Autodesk Fusion 360 part; units mm, degrees
(part 7 of 11)
sketch "Sketch4" plane through (0, 0, 25) normal (0, 0, 1) x (1, 0, 0)
  arc A0 (-57.8411, -108.6864) -> (-56.5947, -103.2256) centre (-92.9957, -97.79) ccw
  arc A1 (-55.7092, -102.5555) -> (-56.5947, -103.2256) centre (-55.8097, -103.3428) ccw
  line L0 (-55.7092, -102.5555) -> (-51.5633, -103.0847)
  spline S0 degree 5 poles (-51.5633, -103.0847) (-51.5364, -103.0882) (-51.4825, -103.0942) (-51.4015, -103.1008) (-51.2932, -103.1049) (-51.1576, -103.1037) (-51.0216, -103.0979) (-50.8855, -103.0894) (-50.7494, -103.0794) (-50.6132, -103.0683) (-50.477, -103.0562) (-50.3407, -103.0425) (-50.2045, -103.0269) (-50.0682, -103.009) (-49.9319, -102.9888) (-49.7956, -102.9666) (-49.6594, -102.9427) (-49.5231, -102.9173) (-49.387, -102.8907) (-49.2509, -102.8628) (-49.1148, -102.8337) (-48.9788, -102.8033) (-48.8429, -102.7715) (-48.7071, -102.7383) (-48.5714, -102.7037) (-48.4357, -102.6678) (-48.3001, -102.6307) (-48.1647, -102.5924) (-48.0293, -102.5529) (-47.8941, -102.5123) (-47.759, -102.4706) (-47.624, -102.4278) (-47.4891, -102.3838) (-47.3544, -102.3388) (-47.2198, -102.2926) (-47.0853, -102.2454) (-46.9509, -102.1971) (-46.8168, -102.1477) (-46.6827, -102.0974) (-46.5488, -102.046) (-46.4151, -101.9936) (-46.2815, -101.9403) (-46.1481, -101.886) (-46.0149, -101.8306) (-45.8818, -101.7744) (-45.7489, -101.7171) (-45.6162, -101.659) (-45.4836, -101.5999) (-45.3513, -101.5398) (-45.2191, -101.4789) (-45.0871, -101.417) (-44.9553, -101.3543) (-44.8237, -101.2906) (-44.6923, -101.2261) (-44.5611, -101.1607) (-44.4302, -101.0944) (-44.2994, -101.0273) (-44.1688, -100.9593) (-44.0384, -100.8904) (-43.9083, -100.8207) (-43.7783, -100.7502) (-43.6486, -100.6788) (-43.5191, -100.6067) (-43.3899, -100.5336) (-43.2608, -100.4598) (-43.132, -100.3852) (-43.0035, -100.3098) (-42.8751, -100.2335) (-42.747, -100.1565) (-42.6192, -100.0787) (-42.4916, -100.0001) (-42.3897, -99.9366) (-42.3133, -99.8886) (-42.2625, -99.8565) (-42.2371, -99.8404) knots 0 0 0 0 0 0 0.01428571 0.02857143 0.04285714 0.05714286 0.07142857 0.08571429 0.1 0.11428571 0.12857143 0.14285714 0.15714286 0.17142857 0.18571429 0.2 0.21428571 0.22857143 0.24285714 0.25714286 0.27142857 0.28571429 0.3 0.31428571 0.32857143 0.34285714 0.35714286 0.37142857 0.38571429 0.4 0.41428571 0.42857143 0.44285714 0.45714286 0.47142857 0.48571429 0.5 0.51428571 0.52857143 0.54285714 0.55714286 0.57142857 0.58571429 0.6 0.61428571 0.62857143 0.64285714 0.65714286 0.67142857 0.68571429 0.7 0.71428571 0.72857143 0.74285714 0.75714286 0.77142857 0.78571429 0.8 0.81428571 0.82857143 0.84285714 0.85714286 0.87142857 0.88571429 0.9 0.91428571 0.92857143 0.94285714 0.95714286 0.97142857 0.98571429 1 1 1 1 1 1
  arc A2 (-42.2371, -99.8404) -> (-42.2371, -95.7395) centre (-92.9957, -97.79) ccw
  spline S1 degree 5 poles (-42.2371, -95.7395) (-42.2625, -95.7234) (-42.3133, -95.6913) (-42.3897, -95.6433) (-42.4916, -95.5798) (-42.6192, -95.5012) (-42.747, -95.4234) (-42.8751, -95.3464) (-43.0035, -95.2702) (-43.132, -95.1947) (-43.2608, -95.1201) (-43.3899, -95.0463) (-43.5191, -94.9733) (-43.6486, -94.9011) (-43.7783, -94.8297) (-43.9083, -94.7592) (-44.0384, -94.6895) (-44.1688, -94.6206) (-44.2994, -94.5526) (-44.4302, -94.4855) (-44.5611, -94.4192) (-44.6923, -94.3538) (-44.8237, -94.2893) (-44.9553, -94.2256) (-45.0871, -94.1629) (-45.2191, -94.101) (-45.3513, -94.0401) (-45.4836, -93.9801) (-45.6162, -93.9209) (-45.7489, -93.8628) (-45.8818, -93.8055) (-46.0149, -93.7493) (-46.1481, -93.694) (-46.2815, -93.6396) (-46.4151, -93.5863) (-46.5488, -93.5339) (-46.6827, -93.4825) (-46.8168, -93.4322) (-46.9509, -93.3829) (-47.0853, -93.3346) (-47.2198, -93.2873) (-47.3544, -93.2411) (-47.4891, -93.1961) (-47.624, -93.1521) (-47.759, -93.1093) (-47.8941, -93.0676) (-48.0293, -93.027) (-48.1647, -92.9875) (-48.3001, -92.9492) (-48.4357, -92.9121) (-48.5714, -92.8762) (-48.7071, -92.8416) (-48.8429, -92.8084) (-48.9788, -92.7766) (-49.1148, -92.7462) (-49.2509, -92.7171) (-49.387, -92.6892) (-49.5231, -92.6626) (-49.6594, -92.6372) (-49.7956, -92.6133) (-49.9319, -92.5911) (-50.0682, -92.5709) (-50.2045, -92.553) (-50.3407, -92.5374) (-50.477, -92.5237) (-50.6132, -92.5116) (-50.7494, -92.5005) (-50.8855, -92.4905) (-51.0216, -92.482) (-51.1576, -92.4762) (-51.2932, -92.475) (-51.4015, -92.4791) (-51.4825, -92.4857) (-51.5364, -92.4917) (-51.5633, -92.4952) knots -1 -1 -1 -1 -1 -1 -0.98571429 -0.97142857 -0.95714286 -0.94285714 -0.92857143 -0.91428571 -0.9 -0.88571429 -0.87142857 -0.85714286 -0.84285714 -0.82857143 -0.81428571 -0.8 -0.78571429 -0.77142857 -0.75714286 -0.74285714 -0.72857143 -0.71428571 -0.7 -0.68571429 -0.67142857 -0.65714286 -0.64285714 -0.62857143 -0.61428571 -0.6 -0.58571429 -0.57142857 -0.55714286 -0.54285714 -0.52857143 -0.51428571 -0.5 -0.48571429 -0.47142857 -0.45714286 -0.44285714 -0.42857143 -0.41428571 -0.4 -0.38571429 -0.37142857 -0.35714286 -0.34285714 -0.32857143 -0.31428571 -0.3 -0.28571429 -0.27142857 -0.25714286 -0.24285714 -0.22857143 -0.21428571 -0.2 -0.18571429 -0.17142857 -0.15714286 -0.14285714 -0.12857143 -0.11428571 -0.1 -0.08571429 -0.07142857 -0.05714286 -0.04285714 -0.02857143 -0.01428571 0 0 0 0 0 0
  line L1 (-51.5633, -92.4952) -> (-55.7092, -93.0245)
  arc A3 (-56.5947, -92.3543) -> (-55.7092, -93.0245) centre (-55.8097, -92.2371) ccw
  arc A4 (-56.5947, -92.3543) -> (-57.8411, -86.8935) centre (-92.9957, -97.79) ccw
  arc A5 (-57.334, -85.9055) -> (-57.8411, -86.8935) centre (-57.083, -86.6585) ccw
  line L2 (-57.334, -85.9055) -> (-53.3691, -84.5835)
  spline S2 degree 5 poles (-53.3691, -84.5835) (-53.3434, -84.575) (-53.2922, -84.557) (-53.2163, -84.5278) (-53.117, -84.4846) (-52.9953, -84.4246) (-52.8753, -84.3604) (-52.7564, -84.2937) (-52.6381, -84.2256) (-52.5202, -84.1565) (-52.4027, -84.0865) (-52.2859, -84.0151) (-52.1699, -83.9418) (-52.0549, -83.8666) (-51.9409, -83.7893) (-51.8277, -83.7102) (-51.7153, -83.6295) (-51.6036, -83.5475) (-51.4925, -83.4644) (-51.3819, -83.3803) (-51.272, -83.295) (-51.1627, -83.2086) (-51.054, -83.121) (-50.9461, -83.0321) (-50.8388, -82.9421) (-50.7321, -82.8509) (-50.6261, -82.7586) (-50.5207, -82.6653) (-50.4158, -82.5711) (-50.3116, -82.4758) (-50.208, -82.3796) (-50.1049, -82.2824) (-50.0025, -82.1843) (-49.9006, -82.0853) (-49.7994, -81.9853) (-49.6987, -81.8843) (-49.5986, -81.7825) (-49.4991, -81.6799) (-49.4002, -81.5763) (-49.3019, -81.472) (-49.2041, -81.3668) (-49.1069, -81.2608) (-49.0103, -81.1539) (-48.9143, -81.0463) (-48.8188, -80.9378) (-48.7239, -80.8286) (-48.6295, -80.7186) (-48.5358, -80.6078) (-48.4426, -80.4963) (-48.3499, -80.3841) (-48.2578, -80.2711) (-48.1663, -80.1574) (-48.0754, -80.0429) (-47.985, -79.9278) (-47.8952, -79.8119) (-47.8059, -79.6954) (-47.7172, -79.5781) (-47.6291, -79.4602) (-47.5415, -79.3416) (-47.4545, -79.2224) (-47.368, -79.1024) (-47.2821, -78.9819) (-47.1967, -78.8606) (-47.112, -78.7388) (-47.0277, -78.6163) (-46.9441, -78.4931) (-46.8609, -78.3694) (-46.7784, -78.245) (-46.6964, -78.1201) (-46.615, -77.9945) (-46.5341, -77.8683) (-46.4698, -77.7669) (-46.4219, -77.6905) (-46.39, -77.6395) (-46.3741, -77.614) knots 0 0 0 0 0 0 0.01428571 0.02857143 0.04285714 0.05714286 0.07142857 0.08571429 0.1 0.11428571 0.12857143 0.14285714 0.15714286 0.17142857 0.18571429 0.2 0.21428571 0.22857143 0.24285714 0.25714286 0.27142857 0.28571429 0.3 0.31428571 0.32857143 0.34285714 0.35714286 0.37142857 0.38571429 0.4 0.41428571 0.42857143 0.44285714 0.45714286 0.47142857 0.48571429 0.5 0.51428571 0.52857143 0.54285714 0.55714286 0.57142857 0.58571429 0.6 0.61428571 0.62857143 0.64285714 0.65714286 0.67142857 0.68571429 0.7 0.71428571 0.72857143 0.74285714 0.75714286 0.77142857 0.78571429 0.8 0.81428571 0.82857143 0.84285714 0.85714286 0.87142857 0.88571429 0.9 0.91428571 0.92857143 0.94285714 0.95714286 0.97142857 0.98571429 1 1 1 1 1 1
  arc A6 (-46.3741, -77.614) -> (-48.1534, -73.9192) centre (-92.9957, -97.79) ccw
  spline S3 degree 5 poles (-48.1534, -73.9192) (-48.1833, -73.9158) (-48.2431, -73.9089) (-48.3326, -73.8987) (-48.452, -73.8857) (-48.6011, -73.8703) (-48.75, -73.8557) (-48.8988, -73.8419) (-49.0475, -73.8289) (-49.1961, -73.8167) (-49.3445, -73.8053) (-49.4928, -73.7948) (-49.641, -73.7851) (-49.789, -73.7763) (-49.9368, -73.7682) (-50.0845, -73.7611) (-50.232, -73.7547) (-50.3793, -73.7493) (-50.5264, -73.7447) (-50.6734, -73.7409) (-50.8202, -73.738) (-50.9668, -73.736) (-51.1132, -73.7349) (-51.2593, -73.7347) (-51.4053, -73.7353) (-51.5511, -73.7369) (-51.6966, -73.7393) (-51.8419, -73.7426) (-51.9869, -73.7469) (-52.1318, -73.7521) (-52.2763, -73.7582) (-52.4206, -73.7652) (-52.5647, -73.7732) (-52.7085, -73.7821) (-52.8519, -73.792) (-52.9951, -73.8028) (-53.1381, -73.8147) (-53.2807, -73.8274) (-53.423, -73.8412) (-53.565, -73.856) (-53.7066, -73.8718) (-53.8479, -73.8886) (-53.9889, -73.9064) (-54.1295, -73.9254) (-54.2697, -73.9453) (-54.4095, -73.9664) (-54.549, -73.9885) (-54.6881, -74.0117) (-54.8267, -74.0359) (-54.965, -74.0613) (-55.1028, -74.0878) (-55.2401, -74.1155) (-55.3768, -74.1446) (-55.5131, -74.1749) (-55.6488, -74.2065) (-55.784, -74.2393) (-55.9187, -74.2732) (-56.053, -74.3083) (-56.1867, -74.3446) (-56.3198, -74.3821) (-56.4523, -74.4213) (-56.5838, -74.4622) (-56.7144, -74.5052) (-56.8439, -74.5502) (-56.9726, -74.597) (-57.1006, -74.6452) (-57.2281, -74.6943) (-57.3551, -74.7444) (-57.4814, -74.7958) (-57.6064, -74.8496) (-57.7292, -74.9073) (-57.8249, -74.958) (-57.895, -74.9991) (-57.941, -75.0279) (-57.9637, -75.0427) knots -1 -1 -1 -1 -1 -1 -0.98571429 -0.97142857 -0.95714286 -0.94285714 -0.92857143 -0.91428571 -0.9 -0.88571429 -0.87142857 -0.85714286 -0.84285714 -0.82857143 -0.81428571 -0.8 -0.78571429 -0.77142857 -0.75714286 -0.74285714 -0.72857143 -0.71428571 -0.7 -0.68571429 -0.67142857 -0.65714286 -0.64285714 -0.62857143 -0.61428571 -0.6 -0.58571429 -0.57142857 -0.55714286 -0.54285714 -0.52857143 -0.51428571 -0.5 -0.48571429 -0.47142857 -0.45714286 -0.44285714 -0.42857143 -0.41428571 -0.4 -0.38571429 -0.37142857 -0.35714286 -0.34285714 -0.32857143 -0.31428571 -0.3 -0.28571429 -0.27142857 -0.25714286 -0.24285714 -0.22857143 -0.21428571 -0.2 -0.18571429 -0.17142857 -0.15714286 -0.14285714 -0.12857143 -0.11428571 -0.1 -0.08571429 -0.07142857 -0.05714286 -0.04285714 -0.02857143 -0.01428571 0 0 0 0 0 0
  line L3 (-57.9637, -75.0427) -> (-61.4694, -77.3184)
  arc A7 (-62.558, -77.0988) -> (-61.4694, -77.3184) centre (-61.9015, -76.6526) ccw
  arc A8 (-62.558, -77.0988) -> (-66.0503, -72.7196) centre (-92.9957, -97.79) ccw
  arc A9 (-66.0221, -71.6094) -> (-66.0503, -72.7196) centre (-65.4692, -72.1789) ccw
  line L4 (-66.0221, -71.6094) -> (-63.0234, -68.698)
  spline S4 degree 5 poles (-63.0234, -68.698) (-63.0039, -68.6791) (-62.9656, -68.6408) (-62.9099, -68.5816) (-62.8392, -68.4995) (-62.7556, -68.3926) (-62.6754, -68.2827) (-62.5972, -68.171) (-62.5201, -68.0583) (-62.4438, -67.945) (-62.3684, -67.8309) (-62.2941, -67.7159) (-62.2214, -67.5996) (-62.1505, -67.4819) (-62.0812, -67.3627) (-62.0136, -67.2424) (-61.9474, -67.1209) (-61.8823, -66.9986) (-61.8182, -66.8755) (-61.7551, -66.7517) (-61.6931, -66.6272) (-61.6321, -66.5019) (-61.5722, -66.3759) (-61.5135, -66.249) (-61.4558, -66.1213) (-61.3993, -65.9928) (-61.3438, -65.8637) (-61.2893, -65.7339) (-61.2358, -65.6035) (-61.1832, -65.4724) (-61.1316, -65.3408) (-61.0809, -65.2085) (-61.0312, -65.0757) (-60.9824, -64.9422) (-60.9346, -64.8082) (-60.8877, -64.6736) (-60.8417, -64.5385) (-60.7966, -64.4028) (-60.7524, -64.2666) (-60.709, -64.1299) (-60.6666, -63.9927) (-60.625, -63.855) (-60.5843, -63.7168) (-60.5445, -63.5782) (-60.5055, -63.4391) (-60.4674, -63.2995) (-60.4302, -63.1594) (-60.3937, -63.019) (-60.3581, -62.878) (-60.3234, -62.7367) (-60.2894, -62.595) (-60.2563, -62.4528) (-60.224, -62.3102) (-60.1926, -62.1673) (-60.1619, -62.0239) (-60.132, -61.8802) (-60.103, -61.7361) (-60.0747, -61.5916) (-60.0473, -61.4467) (-60.0206, -61.3015) (-59.9948, -61.1559) (-59.9697, -61.01) (-59.9454, -60.8638) (-59.9219, -60.7172) (-59.8991, -60.5703) (-59.8772, -60.423) (-59.856, -60.2755) (-59.8356, -60.1276) (-59.8159, -59.9795) (-59.797, -59.831) (-59.7789, -59.6822) (-59.765, -59.563) (-59.755, -59.4734) (-59.7484, -59.4136) (-59.7452, -59.3837) knots 0 0 0 0 0 0 0.01428571 0.02857143 0.04285714 0.05714286 0.07142857 0.08571429 0.1 0.11428571 0.12857143 0.14285714 0.15714286 0.17142857 0.18571429 0.2 0.21428571 0.22857143 0.24285714 0.25714286 0.27142857 0.28571429 0.3 0.31428571 0.32857143 0.34285714 0.35714286 0.37142857 0.38571429 0.4 0.41428571 0.42857143 0.44285714 0.45714286 0.47142857 0.48571429 0.5 0.51428571 0.52857143 0.54285714 0.55714286 0.57142857 0.58571429 0.6 0.61428571 0.62857143 0.64285714 0.65714286 0.67142857 0.68571429 0.7 0.71428571 0.72857143 0.74285714 0.75714286 0.77142857 0.78571429 0.8 0.81428571 0.82857143 0.84285714 0.85714286 0.87142857 0.88571429 0.9 0.91428571 0.92857143 0.94285714 0.95714286 0.97142857 0.98571429 1 1 1 1 1 1
  arc A10 (-59.7452, -59.3837) -> (-62.9513, -56.8269) centre (-92.9957, -97.79) ccw
  spline S5 degree 5 poles (-62.9513, -56.8269) (-62.9798, -56.8367) (-63.0366, -56.8564) (-63.1217, -56.8861) (-63.2349, -56.9262) (-63.3759, -56.977) (-63.5164, -57.0284) (-63.6565, -57.0806) (-63.7961, -57.1334) (-63.9352, -57.1869) (-64.0739, -57.241) (-64.2121, -57.2959) (-64.3498, -57.3514) (-64.4869, -57.4077) (-64.6236, -57.4646) (-64.7598, -57.5222) (-64.8954, -57.5805) (-65.0305, -57.6395) (-65.1651, -57.6992) (-65.2991, -57.7596) (-65.4326, -57.8207) (-65.5656, -57.8824) (-65.6979, -57.9449) (-65.8297, -58.0082) (-65.961, -58.0721) (-66.0916, -58.1367) (-66.2217, -58.202) (-66.3511, -58.2681) (-66.48, -58.3349) (-66.6082, -58.4024) (-66.7358, -58.4706) (-66.8628, -58.5395) (-66.9891, -58.6092) (-67.1148, -58.6796) (-67.2398, -58.7508) (-67.3641, -58.8227) (-67.4877, -58.8954) (-67.6106, -58.9688) (-67.7329, -59.0429) (-67.8544, -59.1178) (-67.9752, -59.1935) (-68.0952, -59.27) (-68.2145, -59.3472) (-68.3329, -59.4253) (-68.4506, -59.5041) (-68.5674, -59.5837) (-68.6835, -59.6642) (-68.7987, -59.7454) (-68.9131, -59.8274) (-69.0267, -59.9102) (-69.1393, -59.9939) (-69.251, -60.0785) (-69.3616, -60.164) (-69.4712, -60.2504) (-69.5798, -60.3378) (-69.6874, -60.426) (-69.794, -60.515) (-69.8997, -60.6049) (-70.0045, -60.6955) (-70.1082, -60.7872) (-70.2105, -60.8799) (-70.3112, -60.9739) (-70.4102, -61.0692) (-70.5074, -61.166) (-70.603, -61.264) (-70.6974, -61.3629) (-70.791, -61.4625) (-70.8837, -61.5628) (-70.9752, -61.6638) (-71.0645, -61.7665) (-71.1501, -61.8718) (-71.2143, -61.959) (-71.2597, -62.0265) (-71.2886, -62.0724) (-71.3027, -62.0956) knots -1 -1 -1 -1 -1 -1 -0.98571429 -0.97142857 -0.95714286 -0.94285714 -0.92857143 -0.91428571 -0.9 -0.88571429 -0.87142857 -0.85714286 -0.84285714 -0.82857143 -0.81428571 -0.8 -0.78571429 -0.77142857 -0.75714286 -0.74285714 -0.72857143 -0.71428571 -0.7 -0.68571429 -0.67142857 -0.65714286 -0.64285714 -0.62857143 -0.61428571 -0.6 -0.58571429 -0.57142857 -0.55714286 -0.54285714 -0.52857143 -0.51428571 -0.5 -0.48571429 -0.47142857 -0.45714286 -0.44285714 -0.42857143 -0.41428571 -0.4 -0.38571429 -0.37142857 -0.35714286 -0.34285714 -0.32857143 -0.31428571 -0.3 -0.28571429 -0.27142857 -0.25714286 -0.24285714 -0.22857143 -0.21428571 -0.2 -0.18571429 -0.17142857 -0.15714286 -0.14285714 -0.12857143 -0.11428571 -0.1 -0.08571429 -0.07142857 -0.05714286 -0.04285714 -0.02857143 -0.01428571 0 0 0 0 0 0
  line L5 (-71.3027, -62.0956) -> (-73.4737, -65.6669)
  arc A11 (-74.5498, -65.9415) -> (-73.4737, -65.6669) centre (-74.152, -65.2546) ccw
  arc A12 (-74.5498, -65.9415) -> (-79.5964, -63.5111) centre (-92.9957, -97.79) ccw
  arc A13 (-80.0527, -62.4987) -> (-79.5964, -63.5111) centre (-79.3074, -62.7719) ccw
  line L6 (-80.0527, -62.4987) -> (-78.6141, -58.5746)
  spline S6 degree 5 poles (-78.6141, -58.5746) (-78.6048, -58.5491) (-78.5869, -58.4979) (-78.5624, -58.4204) (-78.5343, -58.3157) (-78.5053, -58.1832) (-78.4807, -58.0494) (-78.4588, -57.9148) (-78.4382, -57.7798) (-78.4187, -57.6446) (-78.4002, -57.5091) (-78.3832, -57.3732) (-78.3681, -57.2369) (-78.3553, -57.1001) (-78.3446, -56.9627) (-78.3359, -56.8249) (-78.3289, -56.6867) (-78.3234, -56.5483) (-78.319, -56.4096) (-78.3159, -56.2707) (-78.314, -56.1316) (-78.3134, -55.9922) (-78.3142, -55.8527) (-78.3163, -55.7129) (-78.3198, -55.5728) (-78.3246, -55.4326) (-78.3306, -55.2922) (-78.3379, -55.1516) (-78.3462, -55.0108) (-78.3557, -54.87) (-78.3663, -54.7289) (-78.378, -54.5878) (-78.3908, -54.4465) (-78.4048, -54.3051) (-78.4199, -54.1636) (-78.436, -54.022) (-78.4532, -53.8803) (-78.4714, -53.7385) (-78.4907, -53.5966) (-78.511, -53.4546) (-78.5323, -53.3126) (-78.5546, -53.1705) (-78.5778, -53.0284) (-78.6021, -52.8862) (-78.6274, -52.7439) (-78.6536, -52.6016) (-78.6808, -52.4593) (-78.7089, -52.3169) (-78.738, -52.1745) (-78.768, -52.0321) (-78.7989, -51.8896) (-78.8308, -51.7472) (-78.8635, -51.6047) (-78.8972, -51.4623) (-78.9318, -51.3198) (-78.9672, -51.1773) (-79.0036, -51.0349) (-79.0408, -50.8925) (-79.079, -50.75) (-79.1179, -50.6076) (-79.1578, -50.4653) (-79.1985, -50.3229) (-79.2401, -50.1806) (-79.2825, -50.0384) (-79.3257, -49.8961) (-79.3698, -49.7539) (-79.4148, -49.6118) (-79.4605, -49.4697) (-79.5071, -49.3277) (-79.5545, -49.1857) (-79.6027, -49.0438) (-79.642, -48.9304) (-79.6718, -48.8453) (-79.6918, -48.7886) (-79.7018, -48.7602) knots 0 0 0 0 0 0 0.01428571 0.02857143 0.04285714 0.05714286 0.07142857 0.08571429 0.1 0.11428571 0.12857143 0.14285714 0.15714286 0.17142857 0.18571429 0.2 0.21428571 0.22857143 0.24285714 0.25714286 0.27142857 0.28571429 0.3 0.31428571 0.32857143 0.34285714 0.35714286 0.37142857 0.38571429 0.4 0.41428571 0.42857143 0.44285714 0.45714286 0.47142857 0.48571429 0.5 0.51428571 0.52857143 0.54285714 0.55714286 0.57142857 0.58571429 0.6 0.61428571 0.62857143 0.64285714 0.65714286 0.67142857 0.68571429 0.7 0.71428571 0.72857143 0.74285714 0.75714286 0.77142857 0.78571429 0.8 0.81428571 0.82857143 0.84285714 0.85714286 0.87142857 0.88571429 0.9 0.91428571 0.92857143 0.94285714 0.95714286 0.97142857 0.98571429 1 1 1 1 1 1
  arc A14 (-79.7018, -48.7602) -> (-83.6999, -47.8477) centre (-92.9957, -97.79) ccw
  spline S7 degree 5 poles (-83.6999, -47.8477) (-83.7212, -47.8689) (-83.7639, -47.9113) (-83.8276, -47.975) (-83.9122, -48.0602) (-84.0172, -48.1672) (-84.1215, -48.2745) (-84.2251, -48.3822) (-84.328, -48.4904) (-84.4302, -48.599) (-84.5316, -48.7079) (-84.6323, -48.8173) (-84.7322, -48.9271) (-84.8314, -49.0373) (-84.9299, -49.1478) (-85.0275, -49.2588) (-85.1244, -49.3702) (-85.2206, -49.482) (-85.3159, -49.5942) (-85.4105, -49.7067) (-85.5042, -49.8197) (-85.5972, -49.933) (-85.6894, -50.0468) (-85.7807, -50.1609) (-85.8712, -50.2754) (-85.9609, -50.3903) (-86.0497, -50.5056) (-86.1377, -50.6213) (-86.2248, -50.7374) (-86.311, -50.8538) (-86.3964, -50.9707) (-86.4809, -51.0879) (-86.5645, -51.2055) (-86.6471, -51.3235) (-86.7288, -51.4418) (-86.8097, -51.5605) (-86.8895, -51.6796) (-86.9684, -51.7991) (-87.0464, -51.9189) (-87.1234, -52.0392) (-87.1994, -52.1598) (-87.2743, -52.2807) (-87.3482, -52.4021) (-87.4211, -52.5238) (-87.4929, -52.6459) (-87.5636, -52.7683) (-87.6333, -52.8911) (-87.7019, -53.0143) (-87.7694, -53.1378) (-87.8358, -53.2617) (-87.9009, -53.386) (-87.9649, -53.5106) (-88.0274, -53.6357) (-88.0887, -53.7611) (-88.1486, -53.8869) (-88.2072, -54.013) (-88.2647, -54.1395) (-88.321, -54.2664) (-88.376, -54.3935) (-88.4297, -54.5211) (-88.4816, -54.649) (-88.5316, -54.7774) (-88.5794, -54.9063) (-88.625, -55.0356) (-88.6686, -55.1654) (-88.7108, -55.2955) (-88.7518, -55.4258) (-88.7919, -55.5563) (-88.8305, -55.6871) (-88.8664, -55.8184) (-88.8978, -55.9504) (-88.9178, -56.0568) (-88.9294, -56.1372) (-88.9355, -56.1911) (-88.9382, -56.2182) knots -1 -1 -1 -1 -1 -1 -0.98571429 -0.97142857 -0.95714286 -0.94285714 -0.92857143 -0.91428571 -0.9 -0.88571429 -0.87142857 -0.85714286 -0.84285714 -0.82857143 -0.81428571 -0.8 -0.78571429 -0.77142857 -0.75714286 -0.74285714 -0.72857143 -0.71428571 -0.7 -0.68571429 -0.67142857 -0.65714286 -0.64285714 -0.62857143 -0.61428571 -0.6 -0.58571429 -0.57142857 -0.55714286 -0.54285714 -0.52857143 -0.51428571 -0.5 -0.48571429 -0.47142857 -0.45714286 -0.44285714 -0.42857143 -0.41428571 -0.4 -0.38571429 -0.37142857 -0.35714286 -0.34285714 -0.32857143 -0.31428571 -0.3 -0.28571429 -0.27142857 -0.25714286 -0.24285714 -0.22857143 -0.21428571 -0.2 -0.18571429 -0.17142857 -0.15714286 -0.14285714 -0.12857143 -0.11428571 -0.1 -0.08571429 -0.07142857 -0.05714286 -0.04285714 -0.02857143 -0.01428571 0 0 0 0 0 0
  line L7 (-88.9382, -56.2182) -> (-89.3447, -60.3778)
  arc A15 (-90.1951, -61.0921) -> (-89.3447, -60.3778) centre (-90.1347, -60.3006) ccw
  arc A16 (-90.1951, -61.0921) -> (-95.7964, -61.0921) centre (-92.9957, -97.79) ccw
  arc A17 (-96.6467, -60.3778) -> (-95.7964, -61.0921) centre (-95.8568, -60.3006) ccw
  line L8 (-96.6467, -60.3778) -> (-97.0533, -56.2182)
  spline S8 degree 5 poles (-97.0533, -56.2182) (-97.0559, -56.1911) (-97.062, -56.1372) (-97.0736, -56.0568) (-97.0937, -55.9504) (-97.1251, -55.8184) (-97.161, -55.6871) (-97.1996, -55.5563) (-97.2396, -55.4258) (-97.2807, -55.2955) (-97.3228, -55.1654) (-97.3665, -55.0356) (-97.412, -54.9063) (-97.4598, -54.7774) (-97.5098, -54.649) (-97.5618, -54.5211) (-97.6154, -54.3935) (-97.6705, -54.2664) (-97.7268, -54.1395) (-97.7842, -54.013) (-97.8428, -53.8869) (-97.9028, -53.7611) (-97.964, -53.6357) (-98.0266, -53.5106) (-98.0905, -53.386) (-98.1557, -53.2617) (-98.222, -53.1378) (-98.2895, -53.0143) (-98.3581, -52.8911) (-98.4278, -52.7683) (-98.4985, -52.6459) (-98.5703, -52.5238) (-98.6432, -52.4021) (-98.7171, -52.2807) (-98.7921, -52.1598) (-98.8681, -52.0392) (-98.945, -51.9189) (-99.023, -51.7991) (-99.1019, -51.6796) (-99.1818, -51.5605) (-99.2626, -51.4418) (-99.3443, -51.3235) (-99.427, -51.2055) (-99.5106, -51.0879) (-99.595, -50.9707) (-99.6804, -50.8538) (-99.7666, -50.7374) (-99.8538, -50.6213) (-99.9417, -50.5056) (-100.0306, -50.3903) (-100.1202, -50.2754) (-100.2107, -50.1609) (-100.3021, -50.0468) (-100.3942, -49.933) (-100.4872, -49.8197) (-100.581, -49.7067) (-100.6755, -49.5942) (-100.7709, -49.482) (-100.867, -49.3702) (-100.9639, -49.2588) (-101.0616, -49.1478) (-101.16, -49.0373) (-101.2592, -48.9271) (-101.3592, -48.8173) (-101.4599, -48.7079) (-101.5613, -48.599) (-101.6634, -48.4904) (-101.7663, -48.3822) (-101.8699, -48.2745) (-101.9742, -48.1672) (-102.0792, -48.0602) (-102.1638, -47.975) (-102.2275, -47.9113) (-102.2702, -47.8689) (-102.2915, -47.8477) knots 0 0 0 0 0 0 0.01428571 0.02857143 0.04285714 0.05714286 0.07142857 0.08571429 0.1 0.11428571 0.12857143 0.14285714 0.15714286 0.17142857 0.18571429 0.2 0.21428571 0.22857143 0.24285714 0.25714286 0.27142857 0.28571429 0.3 0.31428571 0.32857143 0.34285714 0.35714286 0.37142857 0.38571429 0.4 0.41428571 0.42857143 0.44285714 0.45714286 0.47142857 0.48571429 0.5 0.51428571 0.52857143 0.54285714 0.55714286 0.57142857 0.58571429 0.6 0.61428571 0.62857143 0.64285714 0.65714286 0.67142857 0.68571429 0.7 0.71428571 0.72857143 0.74285714 0.75714286 0.77142857 0.78571429 0.8 0.81428571 0.82857143 0.84285714 0.85714286 0.87142857 0.88571429 0.9 0.91428571 0.92857143 0.94285714 0.95714286 0.97142857 0.98571429 1 1 1 1 1 1
  arc A18 (-102.2915, -47.8477) -> (-106.2896, -48.7602) centre (-92.9957, -97.79) ccw
  spline S9 degree 5 poles (-106.2896, -48.7602) (-106.2996, -48.7886) (-106.3197, -48.8453) (-106.3495, -48.9304) (-106.3887, -49.0438) (-106.4369, -49.1857) (-106.4843, -49.3277) (-106.5309, -49.4697) (-106.5767, -49.6118) (-106.6216, -49.7539) (-106.6657, -49.8961) (-106.709, -50.0384) (-106.7514, -50.1806) (-106.7929, -50.3229) (-106.8336, -50.4653) (-106.8735, -50.6076) (-106.9125, -50.75) (-106.9506, -50.8925) (-106.9878, -51.0349) (-107.0242, -51.1773) (-107.0597, -51.3198) (-107.0942, -51.4623) (-107.1279, -51.6047) (-107.1607, -51.7472) (-107.1925, -51.8896) (-107.2235, -52.0321) (-107.2535, -52.1745) (-107.2825, -52.3169) (-107.3107, -52.4593) (-107.3378, -52.6016) (-107.3641, -52.7439) (-107.3893, -52.8862) (-107.4136, -53.0284) (-107.4369, -53.1705) (-107.4592, -53.3126) (-107.4805, -53.4546) (-107.5007, -53.5966) (-107.52, -53.7385) (-107.5383, -53.8803) (-107.5554, -54.022) (-107.5716, -54.1636) (-107.5866, -54.3051) (-107.6006, -54.4465) (-107.6134, -54.5878) (-107.6251, -54.7289) (-107.6357, -54.87) (-107.6452, -55.0108) (-107.6536, -55.1516) (-107.6608, -55.2922) (-107.6668, -55.4326) (-107.6716, -55.5728) (-107.6751, -55.7129) (-107.6773, -55.8527) (-107.678, -55.9922) (-107.6774, -56.1316) (-107.6755, -56.2707) (-107.6724, -56.4096) (-107.6681, -56.5483) (-107.6625, -56.6867) (-107.6555, -56.8249) (-107.6468, -56.9627) (-107.6361, -57.1001) (-107.6233, -57.2369) (-107.6082, -57.3732) (-107.5912, -57.5091) (-107.5728, -57.6446) (-107.5532, -57.7798) (-107.5327, -57.9148) (-107.5107, -58.0494) (-107.4861, -58.1832) (-107.4571, -58.3157) (-107.429, -58.4204) (-107.4046, -58.4979) (-107.3867, -58.5491) (-107.3773, -58.5746) knots -1 -1 -1 -1 -1 -1 -0.98571429 -0.97142857 -0.95714286 -0.94285714 -0.92857143 -0.91428571 -0.9 -0.88571429 -0.87142857 -0.85714286 -0.84285714 -0.82857143 -0.81428571 -0.8 -0.78571429 -0.77142857 -0.75714286 -0.74285714 -0.72857143 -0.71428571 -0.7 -0.68571429 -0.67142857 -0.65714286 -0.64285714 -0.62857143 -0.61428571 -0.6 -0.58571429 -0.57142857 -0.55714286 -0.54285714 -0.52857143 -0.51428571 -0.5 -0.48571429 -0.47142857 -0.45714286 -0.44285714 -0.42857143 -0.41428571 -0.4 -0.38571429 -0.37142857 -0.35714286 -0.34285714 -0.32857143 -0.31428571 -0.3 -0.28571429 -0.27142857 -0.25714286 -0.24285714 -0.22857143 -0.21428571 -0.2 -0.18571429 -0.17142857 -0.15714286 -0.14285714 -0.12857143 -0.11428571 -0.1 -0.08571429 -0.07142857 -0.05714286 -0.04285714 -0.02857143 -0.01428571 0 0 0 0 0 0
  line L9 (-107.3773, -58.5746) -> (-105.9388, -62.4987)
  arc A19 (-106.395, -63.5111) -> (-105.9388, -62.4987) centre (-106.684, -62.7719) ccw
  arc A20 (-106.395, -63.5111) -> (-111.4416, -65.9415) centre (-92.9957, -97.79) ccw
  arc A21 (-112.5177, -65.6669) -> (-111.4416, -65.9415) centre (-111.8394, -65.2546) ccw
  line L10 (-112.5177, -65.6669) -> (-114.6888, -62.0956)
  spline S10 degree 5 poles (-114.6888, -62.0956) (-114.7029, -62.0724) (-114.7318, -62.0265) (-114.7771, -61.959) (-114.8414, -61.8718) (-114.9269, -61.7665) (-115.0162, -61.6638) (-115.1077, -61.5628) (-115.2004, -61.4625) (-115.294, -61.3629) (-115.3884, -61.264) (-115.484, -61.166) (-115.5812, -61.0692) (-115.6802, -60.9739) (-115.7809, -60.8799) (-115.8833, -60.7872) (-115.9869, -60.6955) (-116.0917, -60.6049) (-116.1974, -60.515) (-116.3041, -60.426) (-116.4117, -60.3378) (-116.5202, -60.2504) (-116.6298, -60.164) (-116.7404, -60.0785) (-116.8521, -59.9939) (-116.9647, -59.9102) (-117.0783, -59.8274) (-117.1927, -59.7454) (-117.308, -59.6642) (-117.424, -59.5837) (-117.5409, -59.5041) (-117.6585, -59.4253) (-117.777, -59.3472) (-117.8962, -59.27) (-118.0163, -59.1935) (-118.137, -59.1178) (-118.2586, -59.0429) (-118.3808, -58.9688) (-118.5037, -58.8954) (-118.6274, -58.8227) (-118.7517, -58.7508) (-118.8767, -58.6796) (-119.0023, -58.6092) (-119.1287, -58.5395) (-119.2556, -58.4706) (-119.3832, -58.4024) (-119.5115, -58.3349) (-119.6403, -58.2681) (-119.7698, -58.202) (-119.8998, -58.1367) (-120.0305, -58.0721) (-120.1617, -58.0082) (-120.2935, -57.9449) (-120.4259, -57.8824) (-120.5588, -57.8207) (-120.6923, -57.7596) (-120.8264, -57.6992) (-120.9609, -57.6395) (-121.096, -57.5805) (-121.2317, -57.5222) (-121.3678, -57.4646) (-121.5045, -57.4077) (-121.6417, -57.3514) (-121.7794, -57.2959) (-121.9175, -57.241) (-122.0562, -57.1869) (-122.1953, -57.1334) (-122.3349, -57.0806) (-122.475, -57.0284) (-122.6156, -56.977) (-122.7566, -56.9262) (-122.8698, -56.8861) (-122.9548, -56.8564) (-123.0117, -56.8367) (-123.0401, -56.8269) knots 0 0 0 0 0 0 0.01428571 0.02857143 0.04285714 0.05714286 0.07142857 0.08571429 0.1 0.11428571 0.12857143 0.14285714 0.15714286 0.17142857 0.18571429 0.2 0.21428571 0.22857143 0.24285714 0.25714286 0.27142857 0.28571429 0.3 0.31428571 0.32857143 0.34285714 0.35714286 0.37142857 0.38571429 0.4 0.41428571 0.42857143 0.44285714 0.45714286 0.47142857 0.48571429 0.5 0.51428571 0.52857143 0.54285714 0.55714286 0.57142857 0.58571429 0.6 0.61428571 0.62857143 0.64285714 0.65714286 0.67142857 0.68571429 0.7 0.71428571 0.72857143 0.74285714 0.75714286 0.77142857 0.78571429 0.8 0.81428571 0.82857143 0.84285714 0.85714286 0.87142857 0.88571429 0.9 0.91428571 0.92857143 0.94285714 0.95714286 0.97142857 0.98571429 1 1 1 1 1 1
  arc A22 (-123.0401, -56.8269) -> (-126.2463, -59.3837) centre (-92.9957, -97.79) ccw
  spline S11 degree 5 poles (-126.2463, -59.3837) (-126.243, -59.4136) (-126.2365, -59.4734) (-126.2264, -59.563) (-126.2125, -59.6822) (-126.1944, -59.831) (-126.1755, -59.9795) (-126.1559, -60.1276) (-126.1354, -60.2755) (-126.1143, -60.423) (-126.0923, -60.5703) (-126.0696, -60.7172) (-126.046, -60.8638) (-126.0218, -61.01) (-125.9967, -61.1559) (-125.9708, -61.3015) (-125.9441, -61.4467) (-125.9167, -61.5916) (-125.8884, -61.7361) (-125.8594, -61.8802) (-125.8295, -62.0239) (-125.7989, -62.1673) (-125.7674, -62.3102) (-125.7351, -62.4528) (-125.702, -62.595) (-125.6681, -62.7367) (-125.6333, -62.878) (-125.5977, -63.019) (-125.5613, -63.1594) (-125.524, -63.2995) (-125.4859, -63.4391) (-125.4469, -63.5782) (-125.4071, -63.7168) (-125.3664, -63.855) (-125.3248, -63.9927) (-125.2824, -64.1299) (-125.2391, -64.2666) (-125.1949, -64.4028) (-125.1498, -64.5385) (-125.1038, -64.6736) (-125.0569, -64.8082) (-125.009, -64.9422) (-124.9603, -65.0757) (-124.9105, -65.2085) (-124.8598, -65.3408) (-124.8082, -65.4724) (-124.7556, -65.6035) (-124.7021, -65.7339) (-124.6476, -65.8637) (-124.5921, -65.9928) (-124.5356, -66.1213) (-124.478, -66.249) (-124.4193, -66.3759) (-124.3594, -66.5019) (-124.2984, -66.6272) (-124.2363, -66.7517) (-124.1732, -66.8755) (-124.1092, -66.9986) (-124.0441, -67.1209) (-123.9778, -67.2424) (-123.9102, -67.3627) (-123.841, -67.4819) (-123.77, -67.5996) (-123.6973, -67.7159) (-123.623, -67.8309) (-123.5476, -67.945) (-123.4713, -68.0583) (-123.3942, -68.171) (-123.3161, -68.2827) (-123.2358, -68.3926) (-123.1522, -68.4995) (-123.0815, -68.5816) (-123.0258, -68.6408) (-122.9875, -68.6791) (-122.968, -68.698) knots -1 -1 -1 -1 -1 -1 -0.98571429 -0.97142857 -0.95714286 -0.94285714 -0.92857143 -0.91428571 -0.9 -0.88571429 -0.87142857 -0.85714286 -0.84285714 -0.82857143 -0.81428571 -0.8 -0.78571429 -0.77142857 -0.75714286 -0.74285714 -0.72857143 -0.71428571 -0.7 -0.68571429 -0.67142857 -0.65714286 -0.64285714 -0.62857143 -0.61428571 -0.6 -0.58571429 -0.57142857 -0.55714286 -0.54285714 -0.52857143 -0.51428571 -0.5 -0.48571429 -0.47142857 -0.45714286 -0.44285714 -0.42857143 -0.41428571 -0.4 -0.38571429 -0.37142857 -0.35714286 -0.34285714 -0.32857143 -0.31428571 -0.3 -0.28571429 -0.27142857 -0.25714286 -0.24285714 -0.22857143 -0.21428571 -0.2 -0.18571429 -0.17142857 -0.15714286 -0.14285714 -0.12857143 -0.11428571 -0.1 -0.08571429 -0.07142857 -0.05714286 -0.04285714 -0.02857143 -0.01428571 0 0 0 0 0 0
  line L11 (-122.968, -68.698) -> (-119.9693, -71.6094)
  arc A23 (-119.9411, -72.7196) -> (-119.9693, -71.6094) centre (-120.5222, -72.1789) ccw
  arc A24 (-119.9411, -72.7196) -> (-123.4335, -77.0988) centre (-92.9957, -97.79) ccw
  arc A25 (-124.5221, -77.3184) -> (-123.4335, -77.0988) centre (-124.0899, -76.6526) ccw
  line L12 (-124.5221, -77.3184) -> (-128.0277, -75.0427)
  spline S12 degree 5 poles (-128.0277, -75.0427) (-128.0505, -75.0279) (-128.0964, -74.9991) (-128.1665, -74.958) (-128.2623, -74.9073) (-128.385, -74.8496) (-128.51, -74.7958) (-128.6363, -74.7444) (-128.7634, -74.6943) (-128.8909, -74.6452) (-129.0189, -74.597) (-129.1475, -74.5502) (-129.2771, -74.5052) (-129.4076, -74.4622) (-129.5392, -74.4213) (-129.6716, -74.3821) (-129.8047, -74.3446) (-129.9385, -74.3083) (-130.0727, -74.2732) (-130.2075, -74.2393) (-130.3426, -74.2065) (-130.4784, -74.1749) (-130.6146, -74.1446) (-130.7514, -74.1155) (-130.8887, -74.0878) (-131.0265, -74.0613) (-131.1647, -74.0359) (-131.3034, -74.0117) (-131.4425, -73.9885) (-131.5819, -73.9664) (-131.7217, -73.9453) (-131.862, -73.9254) (-132.0025, -73.9064) (-132.1435, -73.8886) (-132.2848, -73.8718) (-132.4265, -73.856) (-132.5685, -73.8412) (-132.7108, -73.8274) (-132.8534, -73.8147) (-132.9963, -73.8028) (-133.1395, -73.792) (-133.283, -73.7821) (-133.4268, -73.7732) (-133.5708, -73.7652) (-133.7151, -73.7582) (-133.8597, -73.7521) (-134.0045, -73.7469) (-134.1496, -73.7426) (-134.2949, -73.7393) (-134.4404, -73.7369) (-134.5861, -73.7353) (-134.7321, -73.7347) (-134.8783, -73.7349) (-135.0247, -73.736) (-135.1712, -73.738) (-135.318, -73.7409) (-135.465, -73.7447) (-135.6121, -73.7493) (-135.7595, -73.7547) (-135.907, -73.7611) (-136.0546, -73.7682) (-136.2025, -73.7763) (-136.3505, -73.7851) (-136.4986, -73.7948) (-136.6469, -73.8053) (-136.7953, -73.8167) (-136.9439, -73.8289) (-137.0926, -73.8419) (-137.2414, -73.8557) (-137.3904, -73.8703) (-137.5394, -73.8857) (-137.6588, -73.8987) (-137.7484, -73.9089) (-137.8081, -73.9158) (-137.838, -73.9192) knots 0 0 0 0 0 0 0.01428571 0.02857143 0.04285714 0.05714286 0.07142857 0.08571429 0.1 0.11428571 0.12857143 0.14285714 0.15714286 0.17142857 0.18571429 0.2 0.21428571 0.22857143 0.24285714 0.25714286 0.27142857 0.28571429 0.3 0.31428571 0.32857143 0.34285714 0.35714286 0.37142857 0.38571429 0.4 0.41428571 0.42857143 0.44285714 0.45714286 0.47142857 0.48571429 0.5 0.51428571 0.52857143 0.54285714 0.55714286 0.57142857 0.58571429 0.6 0.61428571 0.62857143 0.64285714 0.65714286 0.67142857 0.68571429 0.7 0.71428571 0.72857143 0.74285714 0.75714286 0.77142857 0.78571429 0.8 0.81428571 0.82857143 0.84285714 0.85714286 0.87142857 0.88571429 0.9 0.91428571 0.92857143 0.94285714 0.95714286 0.97142857 0.98571429 1 1 1 1 1 1
  arc A26 (-137.838, -73.9192) -> (-139.6173, -77.614) centre (-92.9957, -97.79) ccw
  spline S13 degree 5 poles (-139.6173, -77.614) (-139.6014, -77.6395) (-139.5695, -77.6905) (-139.5216, -77.7669) (-139.4573, -77.8683) (-139.3765, -77.9945) (-139.295, -78.1201) (-139.213, -78.245) (-139.1305, -78.3694) (-139.0474, -78.4931) (-138.9637, -78.6163) (-138.8795, -78.7388) (-138.7947, -78.8606) (-138.7094, -78.9819) (-138.6234, -79.1024) (-138.537, -79.2224) (-138.45, -79.3416) (-138.3624, -79.4602) (-138.2742, -79.5781) (-138.1855, -79.6954) (-138.0963, -79.8119) (-138.0064, -79.9278) (-137.9161, -80.0429) (-137.8251, -80.1574) (-137.7336, -80.2711) (-137.6415, -80.3841) (-137.5489, -80.4963) (-137.4557, -80.6078) (-137.3619, -80.7186) (-137.2676, -80.8286) (-137.1727, -80.9378) (-137.0772, -81.0463) (-136.9811, -81.1539) (-136.8845, -81.2608) (-136.7873, -81.3668) (-136.6896, -81.472) (-136.5912, -81.5763) (-136.4923, -81.6799) (-136.3928, -81.7825) (-136.2927, -81.8843) (-136.1921, -81.9853) (-136.0908, -82.0853) (-135.989, -82.1843) (-135.8865, -82.2824) (-135.7835, -82.3796) (-135.6798, -82.4758) (-135.5756, -82.5711) (-135.4708, -82.6653) (-135.3654, -82.7586) (-135.2593, -82.8509) (-135.1527, -82.9421) (-135.0454, -83.0321) (-134.9374, -83.121) (-134.8288, -83.2086) (-134.7195, -83.295) (-134.6095, -83.3803) (-134.499, -83.4644) (-134.3878, -83.5475) (-134.2761, -83.6295) (-134.1637, -83.7102) (-134.0506, -83.7893) (-133.9365, -83.8666) (-133.8215, -83.9418) (-133.7055, -84.0151) (-133.5887, -84.0865) (-133.4713, -84.1565) (-133.3534, -84.2256) (-133.235, -84.2937) (-133.1161, -84.3604) (-132.9961, -84.4246) (-132.8744, -84.4846) (-132.7751, -84.5278) (-132.6993, -84.557) (-132.6481, -84.575) (-132.6223, -84.5835) knots -1 -1 -1 -1 -1 -1 -0.98571429 -0.97142857 -0.95714286 -0.94285714 -0.92857143 -0.91428571 -0.9 -0.88571429 -0.87142857 -0.85714286 -0.84285714 -0.82857143 -0.81428571 -0.8 -0.78571429 -0.77142857 -0.75714286 -0.74285714 -0.72857143 -0.71428571 -0.7 -0.68571429 -0.67142857 -0.65714286 -0.64285714 -0.62857143 -0.61428571 -0.6 -0.58571429 -0.57142857 -0.55714286 -0.54285714 -0.52857143 -0.51428571 -0.5 -0.48571429 -0.47142857 -0.45714286 -0.44285714 -0.42857143 -0.41428571 -0.4 -0.38571429 -0.37142857 -0.35714286 -0.34285714 -0.32857143 -0.31428571 -0.3 -0.28571429 -0.27142857 -0.25714286 -0.24285714 -0.22857143 -0.21428571 -0.2 -0.18571429 -0.17142857 -0.15714286 -0.14285714 -0.12857143 -0.11428571 -0.1 -0.08571429 -0.07142857 -0.05714286 -0.04285714 -0.02857143 -0.01428571 0 0 0 0 0 0
  line L13 (-132.6223, -84.5835) -> (-128.6574, -85.9055)
  arc A27 (-128.1503, -86.8935) -> (-128.6574, -85.9055) centre (-128.9085, -86.6585) ccw
  arc A28 (-128.1503, -86.8935) -> (-129.3967, -92.3543) centre (-92.9957, -97.79) ccw
  arc A29 (-130.2823, -93.0245) -> (-129.3967, -92.3543) centre (-130.1818, -92.2371) ccw
  line L14 (-130.2823, -93.0245) -> (-134.4281, -92.4952)
  spline S14 degree 5 poles (-134.4281, -92.4952) (-134.455, -92.4917) (-134.5089, -92.4857) (-134.5899, -92.4791) (-134.6982, -92.475) (-134.8339, -92.4762) (-134.9698, -92.482) (-135.1059, -92.4905) (-135.2421, -92.5005) (-135.3783, -92.5116) (-135.5145, -92.5237) (-135.6507, -92.5374) (-135.787, -92.553) (-135.9232, -92.5709) (-136.0595, -92.5911) (-136.1958, -92.6133) (-136.3321, -92.6372) (-136.4683, -92.6626) (-136.6045, -92.6892) (-136.7406, -92.7171) (-136.8766, -92.7462) (-137.0126, -92.7766) (-137.1485, -92.8084) (-137.2843, -92.8416) (-137.4201, -92.8762) (-137.5557, -92.9121) (-137.6913, -92.9492) (-137.8267, -92.9875) (-137.9621, -93.027) (-138.0973, -93.0676) (-138.2325, -93.1093) (-138.3674, -93.1521) (-138.5023, -93.1961) (-138.6371, -93.2411) (-138.7717, -93.2873) (-138.9062, -93.3346) (-139.0405, -93.3829) (-139.1747, -93.4322) (-139.3087, -93.4825) (-139.4426, -93.5339) (-139.5763, -93.5863) (-139.7099, -93.6396) (-139.8433, -93.694) (-139.9766, -93.7493) (-140.1096, -93.8055) (-140.2425, -93.8628) (-140.3752, -93.9209) (-140.5078, -93.9801) (-140.6401, -94.0401) (-140.7723, -94.101) (-140.9043, -94.1629) (-141.0361, -94.2256) (-141.1677, -94.2893) (-141.2991, -94.3538) (-141.4303, -94.4192) (-141.5613, -94.4855) (-141.6921, -94.5526) (-141.8226, -94.6206) (-141.953, -94.6895) (-142.0832, -94.7592) (-142.2131, -94.8297) (-142.3428, -94.9011) (-142.4723, -94.9733) (-142.6016, -95.0463) (-142.7306, -95.1201) (-142.8594, -95.1947) (-142.988, -95.2702) (-143.1163, -95.3464) (-143.2444, -95.4234) (-143.3723, -95.5012) (-143.4999, -95.5798) (-143.6018, -95.6433) (-143.6781, -95.6913) (-143.7289, -95.7234) (-143.7543, -95.7395) knots 0 0 0 0 0 0 0.01428571 0.02857143 0.04285714 0.05714286 0.07142857 0.08571429 0.1 0.11428571 0.12857143 0.14285714 0.15714286 0.17142857 0.18571429 0.2 0.21428571 0.22857143 0.24285714 0.25714286 0.27142857 0.28571429 0.3 0.31428571 0.32857143 0.34285714 0.35714286 0.37142857 0.38571429 0.4 0.41428571 0.42857143 0.44285714 0.45714286 0.47142857 0.48571429 0.5 0.51428571 0.52857143 0.54285714 0.55714286 0.57142857 0.58571429 0.6 0.61428571 0.62857143 0.64285714 0.65714286 0.67142857 0.68571429 0.7 0.71428571 0.72857143 0.74285714 0.75714286 0.77142857 0.78571429 0.8 0.81428571 0.82857143 0.84285714 0.85714286 0.87142857 0.88571429 0.9 0.91428571 0.92857143 0.94285714 0.95714286 0.97142857 0.98571429 1 1 1 1 1 1
  arc A30 (-143.7543, -95.7395) -> (-143.7543, -99.8404) centre (-92.9957, -97.79) ccw
  spline S15 degree 5 poles (-143.7543, -99.8404) (-143.7289, -99.8565) (-143.6781, -99.8886) (-143.6018, -99.9366) (-143.4999, -100.0001) (-143.3723, -100.0787) (-143.2444, -100.1565) (-143.1163, -100.2335) (-142.988, -100.3098) (-142.8594, -100.3852) (-142.7306, -100.4598) (-142.6016, -100.5336) (-142.4723, -100.6067) (-142.3428, -100.6788) (-142.2131, -100.7502) (-142.0832, -100.8207) (-141.953, -100.8904) (-141.8226, -100.9593) (-141.6921, -101.0273) (-141.5613, -101.0944) (-141.4303, -101.1607) (-141.2991, -101.2261) (-141.1677, -101.2906) (-141.0361, -101.3543) (-140.9043, -101.417) (-140.7723, -101.4789) (-140.6401, -101.5398) (-140.5078, -101.5999) (-140.3752, -101.659) (-140.2425, -101.7171) (-140.1096, -101.7744) (-139.9766, -101.8306) (-139.8433, -101.886) (-139.7099, -101.9403) (-139.5763, -101.9936) (-139.4426, -102.046) (-139.3087, -102.0974) (-139.1747, -102.1477) (-139.0405, -102.1971) (-138.9062, -102.2454) (-138.7717, -102.2926) (-138.6371, -102.3388) (-138.5023, -102.3838) (-138.3674, -102.4278) (-138.2325, -102.4706) (-138.0973, -102.5123) (-137.9621, -102.5529) (-137.8267, -102.5924) (-137.6913, -102.6307) (-137.5557, -102.6678) (-137.4201, -102.7037) (-137.2843, -102.7383) (-137.1485, -102.7715) (-137.0126, -102.8033) (-136.8766, -102.8337) (-136.7406, -102.8628) (-136.6045, -102.8907) (-136.4683, -102.9173) (-136.3321, -102.9427) (-136.1958, -102.9666) (-136.0595, -102.9888) (-135.9232, -103.009) (-135.787, -103.0269) (-135.6507, -103.0425) (-135.5145, -103.0562) (-135.3783, -103.0683) (-135.2421, -103.0794) (-135.1059, -103.0894) (-134.9698, -103.0979) (-134.8339, -103.1037) (-134.6982, -103.1049) (-134.5899, -103.1008) (-134.5089, -103.0942) (-134.455, -103.0882) (-134.4281, -103.0847) knots -1 -1 -1 -1 -1 -1 -0.98571429 -0.97142857 -0.95714286 -0.94285714 -0.92857143 -0.91428571 -0.9 -0.88571429 -0.87142857 -0.85714286 -0.84285714 -0.82857143 -0.81428571 -0.8 -0.78571429 -0.77142857 -0.75714286 -0.74285714 -0.72857143 -0.71428571 -0.7 -0.68571429 -0.67142857 -0.65714286 -0.64285714 -0.62857143 -0.61428571 -0.6 -0.58571429 -0.57142857 -0.55714286 -0.54285714 -0.52857143 -0.51428571 -0.5 -0.48571429 -0.47142857 -0.45714286 -0.44285714 -0.42857143 -0.41428571 -0.4 -0.38571429 -0.37142857 -0.35714286 -0.34285714 -0.32857143 -0.31428571 -0.3 -0.28571429 -0.27142857 -0.25714286 -0.24285714 -0.22857143 -0.21428571 -0.2 -0.18571429 -0.17142857 -0.15714286 -0.14285714 -0.12857143 -0.11428571 -0.1 -0.08571429 -0.07142857 -0.05714286 -0.04285714 -0.02857143 -0.01428571 0 0 0 0 0 0
  line L15 (-134.4281, -103.0847) -> (-130.2823, -102.5555)
  arc A31 (-129.3967, -103.2256) -> (-130.2823, -102.5555) centre (-130.1818, -103.3428) ccw
  arc A32 (-129.3967, -103.2256) -> (-128.1503, -108.6864) centre (-92.9957, -97.79) ccw
  arc A33 (-128.6574, -109.6744) -> (-128.1503, -108.6864) centre (-128.9085, -108.9214) ccw
  line L16 (-128.6574, -109.6744) -> (-132.6223, -110.9964)
  spline S16 degree 5 poles (-132.6223, -110.9964) (-132.6481, -111.005) (-132.6993, -111.0229) (-132.7751, -111.0521) (-132.8744, -111.0954) (-132.9961, -111.1553) (-133.1161, -111.2195) (-133.235, -111.2863) (-133.3534, -111.3544) (-133.4713, -111.4234) (-133.5887, -111.4934) (-133.7055, -111.5649) (-133.8215, -111.6381) (-133.9365, -111.7133) (-134.0506, -111.7906) (-134.1637, -111.8698) (-134.2761, -111.9504) (-134.3878, -112.0324) (-134.499, -112.1155) (-134.6095, -112.1997) (-134.7195, -112.2849) (-134.8288, -112.3713) (-134.9374, -112.4589) (-135.0454, -112.5478) (-135.1527, -112.6378) (-135.2593, -112.729) (-135.3654, -112.8213) (-135.4708, -112.9146) (-135.5756, -113.0089) (-135.6798, -113.1041) (-135.7835, -113.2003) (-135.8865, -113.2975) (-135.989, -113.3956) (-136.0908, -113.4947) (-136.1921, -113.5947) (-136.2927, -113.6956) (-136.3928, -113.7974) (-136.4923, -113.9) (-136.5912, -114.0036) (-136.6896, -114.1079) (-136.7873, -114.2131) (-136.8845, -114.3192) (-136.9811, -114.426) (-137.0772, -114.5336) (-137.1727, -114.6421) (-137.2676, -114.7513) (-137.3619, -114.8613) (-137.4557, -114.9721) (-137.5489, -115.0836) (-137.6415, -115.1958) (-137.7336, -115.3088) (-137.8251, -115.4225) (-137.9161, -115.537) (-138.0064, -115.6521) (-138.0963, -115.768) (-138.1855, -115.8845) (-138.2742, -116.0018) (-138.3624, -116.1197) (-138.45, -116.2383) (-138.537, -116.3576) (-138.6234, -116.4775) (-138.7094, -116.5981) (-138.7947, -116.7193) (-138.8795, -116.8412) (-138.9637, -116.9637) (-139.0474, -117.0868) (-139.1305, -117.2105) (-139.213, -117.3349) (-139.295, -117.4599) (-139.3765, -117.5854) (-139.4573, -117.7116) (-139.5216, -117.813) (-139.5695, -117.8894) (-139.6014, -117.9404) (-139.6173, -117.9659) knots 0 0 0 0 0 0 0.01428571 0.02857143 0.04285714 0.05714286 0.07142857 0.08571429 0.1 0.11428571 0.12857143 0.14285714 0.15714286 0.17142857 0.18571429 0.2 0.21428571 0.22857143 0.24285714 0.25714286 0.27142857 0.28571429 0.3 0.31428571 0.32857143 0.34285714 0.35714286 0.37142857 0.38571429 0.4 0.41428571 0.42857143 0.44285714 0.45714286 0.47142857 0.48571429 0.5 0.51428571 0.52857143 0.54285714 0.55714286 0.57142857 0.58571429 0.6 0.61428571 0.62857143 0.64285714 0.65714286 0.67142857 0.68571429 0.7 0.71428571 0.72857143 0.74285714 0.75714286 0.77142857 0.78571429 0.8 0.81428571 0.82857143 0.84285714 0.85714286 0.87142857 0.88571429 0.9 0.91428571 0.92857143 0.94285714 0.95714286 0.97142857 0.98571429 1 1 1 1 1 1
  arc A34 (-139.6173, -117.9659) -> (-137.838, -121.6607) centre (-92.9957, -97.79) ccw
  spline S17 degree 5 poles (-137.838, -121.6607) (-137.8081, -121.6642) (-137.7484, -121.6711) (-137.6588, -121.6812) (-137.5394, -121.6942) (-137.3904, -121.7096) (-137.2414, -121.7242) (-137.0926, -121.738) (-136.9439, -121.751) (-136.7953, -121.7632) (-136.6469, -121.7746) (-136.4986, -121.7851) (-136.3505, -121.7948) (-136.2025, -121.8037) (-136.0546, -121.8117) (-135.907, -121.8188) (-135.7595, -121.8252) (-135.6121, -121.8306) (-135.465, -121.8352) (-135.318, -121.839) (-135.1712, -121.8419) (-135.0247, -121.8439) (-134.8783, -121.845) (-134.7321, -121.8452) (-134.5861, -121.8446) (-134.4404, -121.8431) (-134.2949, -121.8406) (-134.1496, -121.8373) (-134.0045, -121.833) (-133.8597, -121.8278) (-133.7151, -121.8217) (-133.5708, -121.8147) (-133.4268, -121.8067) (-133.283, -121.7978) (-133.1395, -121.7879) (-132.9963, -121.7771) (-132.8534, -121.7653) (-132.7108, -121.7525) (-132.5685, -121.7387) (-132.4265, -121.7239) (-132.2848, -121.7081) (-132.1435, -121.6913) (-132.0025, -121.6735) (-131.862, -121.6546) (-131.7217, -121.6346) (-131.5819, -121.6135) (-131.4425, -121.5914) (-131.3034, -121.5682) (-131.1647, -121.544) (-131.0265, -121.5186) (-130.8887, -121.4921) (-130.7514, -121.4644) (-130.6146, -121.4353) (-130.4784, -121.405) (-130.3426, -121.3734) (-130.2075, -121.3406) (-130.0727, -121.3067) (-129.9385, -121.2716) (-129.8047, -121.2354) (-129.6716, -121.1978) (-129.5392, -121.1587) (-129.4076, -121.1177) (-129.2771, -121.0747) (-129.1475, -121.0297) (-129.0189, -120.9829) (-128.8909, -120.9347) (-128.7634, -120.8856) (-128.6363, -120.8355) (-128.51, -120.7841) (-128.385, -120.7304) (-128.2623, -120.6726) (-128.1665, -120.6219) (-128.0964, -120.5808) (-128.0505, -120.552) (-128.0277, -120.5372) knots -1 -1 -1 -1 -1 -1 -0.98571429 -0.97142857 -0.95714286 -0.94285714 -0.92857143 -0.91428571 -0.9 -0.88571429 -0.87142857 -0.85714286 -0.84285714 -0.82857143 -0.81428571 -0.8 -0.78571429 -0.77142857 -0.75714286 -0.74285714 -0.72857143 -0.71428571 -0.7 -0.68571429 -0.67142857 -0.65714286 -0.64285714 -0.62857143 -0.61428571 -0.6 -0.58571429 -0.57142857 -0.55714286 -0.54285714 -0.52857143 -0.51428571 -0.5 -0.48571429 -0.47142857 -0.45714286 -0.44285714 -0.42857143 -0.41428571 -0.4 -0.38571429 -0.37142857 -0.35714286 -0.34285714 -0.32857143 -0.31428571 -0.3 -0.28571429 -0.27142857 -0.25714286 -0.24285714 -0.22857143 -0.21428571 -0.2 -0.18571429 -0.17142857 -0.15714286 -0.14285714 -0.12857143 -0.11428571 -0.1 -0.08571429 -0.07142857 -0.05714286 -0.04285714 -0.02857143 -0.01428571 0 0 0 0 0 0
  line L17 (-128.0277, -120.5372) -> (-124.5221, -118.2616)
  arc A35 (-123.4335, -118.4811) -> (-124.5221, -118.2616) centre (-124.0899, -118.9273) ccw
  arc A36 (-123.4335, -118.4811) -> (-119.9411, -122.8603) centre (-92.9957, -97.79) ccw
  arc A37 (-119.9693, -123.9705) -> (-119.9411, -122.8603) centre (-120.5222, -123.401) ccw
  line L18 (-119.9693, -123.9705) -> (-122.968, -126.8819)